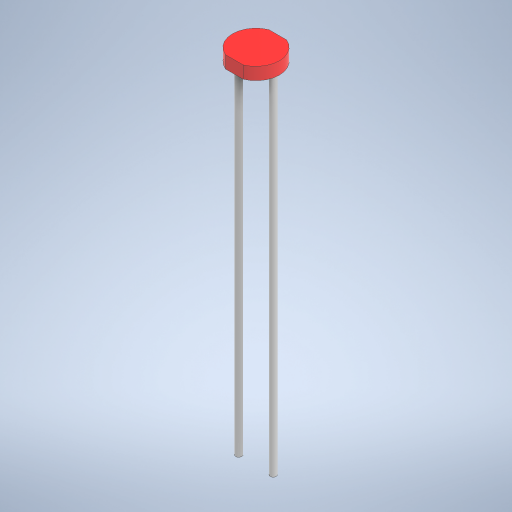
# Autodesk Inventor part: PhotoResistor
Saved by Autodesk Inventor 2023 (Build 270158000, 158)
## iProperties
Created: 2023-09-28
Part Number: PhotoResistor
Material: Generic
Document SubType Name: Modeling
Designer: Gage
Density: 1 g/cm^3
Appearance: Default
Author: Gage
Autodesk Inventor part; units mm, degrees
ref_plane "YZ Plane" through (0, 0, 0) normal (1, 0, 0) x (0, 1, 0)
ref_plane "XZ Plane" through (0, 0, 0) normal (0, 1, 0) x (-1, 0, 0)
ref_plane "XY Plane" through (0, 0, 0) normal (0, 0, 1) x (1, 0, 0)
sketch "Sketch2" plane through (0, 0, 0) normal (0, 1, 0) x (-1, 0, 0)
  line L0 (0.8521, -2.0836) -> (-0.8521, -2.0836)
  line L1 (-0.8521, 2.0836) -> (0.8521, 2.0836)
  arc A0 (0.8521, -2.0836) -> (0.8521, 2.0836) centre (0, 0) ccw
  arc A1 (-0.8521, 2.0836) -> (-0.8521, -2.0836) centre (0, 0) ccw
  point P0 (0, -2.0836)
  constraints: 4 end point, 4 point on circle, 2 centre point, 1 coincident, 1 horizontal, 1 midpoint, 1 parallel, 1 vertical alignment
extrude "Extrusion1" add sketch "Sketch2" along normal blind 1.1906
sketch "Sketch3" plane through (0, 0, 0) normal (0, -1, 0) x (1, 0, 0)
  circle A0 centre (-1.6558, 0) radius 0.2977
  circle A1 centre (1.6558, 0) radius 0.2977
  arc A2 (0.8521, -2.0836) -> (0.8521, 2.0836) centre (0, 0) ccw projected
  arc A3 (-0.8521, 2.0836) -> (-0.8521, -2.0836) centre (0, 0) ccw projected
  point P0 (2.2511, 0)
  point P1 (-2.2511, 0)
  dimension "d6" = 0.5953
  dimension "d7" = 0.5953
  dimension "d8" = 0.5953
  dimension "d9" = 0.5953
  constraints: 2 centre point, 2 point on circle
  measures "d6" diameter of A0
  measures "d7" diameter of A1
  measures "d8" distance of point (2.251, 0) A1.centre
  measures "d9" distance of point (-2.251, 0) A0.centre
extrude "Extrusion2" add sketch "Sketch3" along normal blind 33.5359
body "Solid1"
